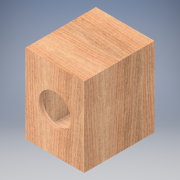
# Autodesk Inventor part: speakerBox
Saved by Autodesk Inventor 2017 (Build 210142000, 142)
## iProperties
Created: 2018-07-22
Part Number: speakerBox
Material: Wood (Birch)
Document SubType Name: Modeling
Designer: Jake
Density: 0.55 g/cm^3
Appearance: Birch - Natural Polished
Author: Jake
Autodesk Inventor part; units mm, degrees
ref_plane "YZ Plane" through (0, 0, 0) normal (1, 0, 0) x (0, 1, 0)
ref_plane "XZ Plane" through (0, 0, 0) normal (0, 1, 0) x (-1, 0, 0)
ref_plane "XY Plane" through (0, 0, 0) normal (0, 0, 1) x (1, 0, 0)
sketch "Sketch1" plane through (0, 0, 0) normal (0, 1, 0) x (-1, 0, 0)
  line L0 (127, 152.4) -> (-127, 152.4)
  line L1 (-127, 152.4) -> (-127, -152.4)
  line L2 (-127, -152.4) -> (127, -152.4)
  line L3 (127, -152.4) -> (127, 152.4)
  point P0 (0, 0)
  point P1 (127, 0)
  point P2 (0, -152.4)
  dimension "d0" = 304.8
  dimension "d1" = 254
  constraints: 8 end point, 2 midpoint, 2 parallel, 1 horizontal, 1 horizontal alignment, 1 perpendicular, 1 vertical alignment
  measures "d0" distance of L2.end L0.start
  measures "d1" distance of L1.end L2.end
extrude "Extrusion1" add sketch "Sketch1" along normal blind 19.05
sketch "Sketch4" plane through (0, 19.05, 0) normal (0, 1, 0) x (1, 0, 0)
  line L0 (-127, -152.4) -> (127, -152.4) projected
  line L1 (127, -152.4) -> (127, 152.4) projected
  line L2 (127, 152.4) -> (-127, 152.4) projected
  line L3 (-127, 152.4) -> (-127, -152.4) projected
  line L4 (-127, -152.4) -> (127, -152.4) projected
  line L5 (-127, -152.4) -> (107.95, -152.4)
  line L6 (107.95, -152.4) -> (107.95, -133.35)
  line L7 (107.95, -133.35) -> (-127, -133.35)
  line L8 (-127, -133.35) -> (-127, -152.4)
  point P0 (0, 0)
  dimension "d4" = 19.05
  dimension "d5" = 19.05
  constraints: 8 end point, 2 parallel, 1 horizontal, 1 perpendicular
  measures "d4" distance between parallel lines of L0 L7
  measures "d5" distance between parallel lines of L1 L6
extrude "Extrusion2" add sketch "Sketch4" along normal blind 304.8 contours L3 L7 L6 L0
sketch "Sketch5" plane through (0, 19.05, 0) normal (0, 1, 0) x (1, 0, 0)
  line L0 (107.95, -133.35) -> (107.95, -152.4) projected
  line L1 (107.95, -152.4) -> (127, -152.4) projected
  line L2 (127, -152.4) -> (127, 152.4) projected
  line L3 (127, 152.4) -> (-127, 152.4) projected
  line L4 (-127, 152.4) -> (-127, -133.35) projected
  line L5 (-127, -133.35) -> (107.95, -133.35) projected
  line L6 (-127, -152.4) -> (127, -152.4) projected
  line L7 (127, -152.4) -> (107.95, -152.4)
  line L8 (107.95, -152.4) -> (107.95, 133.35)
  line L9 (107.95, 133.35) -> (127, 133.35)
  line L10 (127, 133.35) -> (127, -152.4)
  line L11 (107.95, -152.4) -> (107.95, -133.35) projected
  point P0 (0, 0)
  dimension "d8" = 19.05
  constraints: 8 end point, 2 parallel, 1 collinear, 1 horizontal, 1 perpendicular
  measures "d8" distance between parallel lines of L3 L9
extrude "Extrusion3" add sketch "Sketch5" along normal blind 304.8 contours L8 L9 L2 L1 L0
sketch "Sketch6" plane through (0, 19.05, 0) normal (0, 1, 0) x (1, 0, 0)
  line L0 (107.95, 133.35) -> (127, 133.35) projected
  line L1 (127, 133.35) -> (127, 152.4) projected
  line L2 (127, 152.4) -> (-127, 152.4) projected
  line L3 (-127, 152.4) -> (-127, -133.35) projected
  line L4 (-127, -133.35) -> (107.95, -133.35) projected
  line L5 (107.95, -133.35) -> (107.95, 133.35) projected
  line L6 (127, 152.4) -> (-107.95, 152.4)
  line L7 (-107.95, 152.4) -> (-107.95, 133.35)
  line L8 (-107.95, 133.35) -> (127, 133.35)
  line L9 (127, 133.35) -> (127, 152.4)
  line L10 (127, 133.35) -> (107.95, 133.35) projected
  point P0 (0, 0)
  dimension "d11" = 19.05
  constraints: 8 end point, 2 parallel, 1 collinear, 1 horizontal, 1 perpendicular
  measures "d11" distance between parallel lines of L3 L7
extrude "Extrusion4" add sketch "Sketch6" along normal blind 304.8 contours L8 L7 L2 L1 L0
sketch "Sketch7" plane through (0, 19.05, 0) normal (0, 1, 0) x (1, 0, 0)
  line L0 (-107.95, 133.35) -> (-107.95, 152.4) projected
  line L1 (-107.95, 152.4) -> (-127, 152.4) projected
  line L2 (-127, 152.4) -> (-127, -133.35) projected
  line L3 (-127, -133.35) -> (107.95, -133.35) projected
  line L4 (107.95, -133.35) -> (107.95, 133.35) projected
  line L5 (107.95, 133.35) -> (-107.95, 133.35) projected
  line L6 (-127, -133.35) -> (107.95, -133.35) projected
  line L7 (-127, 152.4) -> (-107.95, 152.4)
  line L8 (-107.95, 152.4) -> (-107.95, -133.35)
  line L9 (-107.95, -133.35) -> (-127, -133.35)
  line L10 (-127, -133.35) -> (-127, 152.4)
  line L11 (-107.95, 152.4) -> (-107.95, 133.35) projected
  point P0 (0, 0)
  constraints: 8 end point, 2 parallel, 1 collinear, 1 horizontal, 1 perpendicular, 1 point on line
extrude "Extrusion5" add sketch "Sketch7" along normal blind 304.8 contours L8 L3 L2 L1 L0
sketch "Sketch8" plane through (0, 323.85, 0) normal (0, 1, 0) x (1, 0, 0)
  line L0 (-107.95, 133.35) -> (107.95, 133.35) projected
  line L1 (107.95, 133.35) -> (107.95, -133.35) projected
  line L2 (107.95, -133.35) -> (-107.95, -133.35) projected
  line L3 (-107.95, -133.35) -> (-107.95, 133.35) projected
  line L4 (127, 152.4) -> (-127, 152.4) projected
  line L5 (-127, 152.4) -> (-127, -152.4) projected
  line L6 (-127, -152.4) -> (127, -152.4) projected
  line L7 (127, -152.4) -> (127, 152.4) projected
  line L8 (127, -152.4) -> (127, 152.4) projected
  line L9 (-127, 152.4) -> (127, 152.4)
  line L10 (127, 152.4) -> (127, -152.4)
  line L11 (127, -152.4) -> (-127, -152.4)
  line L12 (-127, -152.4) -> (-127, 152.4)
  point P0 (0, 0)
  constraints: 8 end point, 2 parallel, 1 horizontal, 1 perpendicular
extrude "Extrusion6" add sketch "Sketch8" along normal blind 19.05 contours L0 L1 L2 L3 | L7 L6 L5 L4
sketch "Sketch9" plane through (-127, 0, 152.4) normal (0, 0, 1) x (1, 0, 0)
  circle A0 centre (127, 171.45) radius 69.5
  line L0 (0, 0) -> (254, 0) projected
  line L1 (254, 0) -> (254, 342.9) projected
  line L2 (0, 0) -> (0, 342.9) projected
  line L3 (0, 342.9) -> (254, 342.9) projected
  line L4 (0, 342.9) -> (254, 342.9) projected
  point P0 (127, 0)
  point P1 (254, 171.45)
  point P2 (127, 342.9)
  dimension "d18" = 139
  constraints: 2 midpoint, 1 centre point, 1 horizontal alignment, 1 vertical alignment
  measures "d18" diameter of A0
extrude "Extrusion7" cut sketch "Sketch9" against normal up to next contours A0
sketch "Sketch10" plane through (0, 19.05, 0) normal (0, 1, 0) x (1, 0, 0)
  line L0 (-107.95, 133.35) -> (-107.95, -133.35) projected
  line L1 (-107.95, -133.35) -> (107.95, -133.35) projected
  line L2 (107.95, -133.35) -> (107.95, 133.35) projected
  line L3 (107.95, 133.35) -> (-107.95, 133.35) projected
  line L4 (-107.95, 133.35) -> (-82.55, 133.35)
  line L5 (-82.55, 133.35) -> (-82.55, 107.95)
  line L6 (-82.55, 107.95) -> (-107.95, 107.95)
  line L7 (-107.95, 107.95) -> (-107.95, 133.35)
  line L8 (107.95, 133.35) -> (82.55, 133.35)
  line L9 (82.55, 133.35) -> (82.55, 107.95)
  line L10 (82.55, 107.95) -> (107.95, 107.95)
  line L11 (107.95, 107.95) -> (107.95, 133.35)
  line L12 (-107.95, -133.35) -> (-82.55, -133.35)
  line L13 (-82.55, -133.35) -> (-82.55, -107.95)
  line L14 (-82.55, -107.95) -> (-107.95, -107.95)
  line L15 (-107.95, -107.95) -> (-107.95, -133.35)
  line L16 (107.95, -133.35) -> (82.55, -133.35)
  line L17 (82.55, -133.35) -> (82.55, -107.95)
  line L18 (82.55, -107.95) -> (107.95, -107.95)
  line L19 (107.95, -107.95) -> (107.95, -133.35)
  point P0 (0, 0)
  dimension "d21" = 25.4
  dimension "d22" = 25.4
  dimension "d23" = 25.4
  dimension "d24" = 25.4
  dimension "d25" = 25.4
  dimension "d26" = 25.4
  constraints: 32 end point, 8 parallel, 4 horizontal, 4 perpendicular, 2 point on line
  measures "d21" distance of L4.end L5.end
  measures "d22" distance of L5.end L6.end
  measures "d23" distance of L9.end L10.end
  measures "d24" distance of L13.end L14.end
  measures "d25" distance of L12.end L13.end
  measures "d26" distance of L17.end L18.end
extrude "Extrusion8" add sketch "Sketch10" along normal up to surface (304.8 mm away) contours L3 L5 L6 L0 | L14 L13 L1 L0 | L3 L2 L10 L9 | L17 L18 L2 L1
equation "\"d5\" = d4"
body "Solid1"
